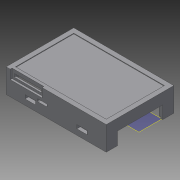
# Autodesk Inventor part: Boden
Saved by Autodesk Inventor 2014 (Build 180170000, 170)
## iProperties
Created: 2016-07-27
Part Number: Boden
Material: Generisch
Document SubType Name: Modeling
Designer: cem
Density: 1 g/cm^3
Appearance: Vorgabe
Author: cem
Autodesk Inventor part; units mm, degrees
ref_plane "YZ Plane" through (0, 0, 0) normal (1, 0, 0) x (0, 1, 0)
ref_plane "XZ Plane" through (0, 0, 0) normal (0, 1, 0) x (-1, 0, 0)
ref_plane "EbeneBoden" through (-11.5031, -4.6031, 1.9) normal (0, 0, 1) x (1, 0, 0)
ref_plane "EbeneWändeEnde" through (17.7, 4.9, -6.9) normal (0, 0, -1) x (-1, 0, 0)
sketch "SkizzeBoden" plane through (-11.5031, -4.6031, 1.9) normal (0, 0, 1) x (1, 0, 0)
  line L0 (-7.1969, 7.4031) -> (6.8031, 7.4031) projected
  line L1 (6.8031, 7.4031) -> (6.8031, -7.7969) projected
  line L2 (6.8031, -7.7969) -> (4.3031, -7.7969) projected
  line L3 (4.3031, -7.7969) -> (4.3031, -6.7969) projected
  line L4 (4.3031, -6.7969) -> (-7.1969, -6.7969) projected
  line L5 (-7.1969, -6.7969) -> (-7.1969, 7.4031) projected
  line L6 (31.5031, 17.6031) -> (-8.4969, 17.6031) projected
  line L7 (-8.4969, 17.6031) -> (-8.4969, -8.3969) projected
  line L8 (-8.4969, -8.3969) -> (31.5031, -8.3969) projected
  line L9 (31.5031, -8.3969) -> (31.5031, 17.6031) projected
  line L10 (-18.7369, 4.6031) -> (41.7431, 4.6031) projected
  line L11 (11.5031, -15.8369) -> (11.5031, 25.0431) projected
  line L12 (-10.0969, 19.2031) -> (33.1031, 19.2031)
  line L13 (33.1031, 19.2031) -> (33.1031, -9.9969)
  line L14 (33.1031, -9.9969) -> (-10.0969, -9.9969)
  line L15 (-10.0969, -9.9969) -> (-10.0969, 19.2031)
  point P0 (11.5031, 4.6031)
  dimension "d0" = 1.6
  constraints: 8 end point, 3 other
  measures "d0" distance between parallel lines of L7 L15
extrude "Boden" add sketch "SkizzeBoden" along normal blind 1.5
sketch "SkizzeWände" plane through (-11.5031, -4.6031, 1.9) normal (0, 0, -1) x (-1, 0, 0)
  line L0 (10.0969, 19.2031) -> (-33.1031, 19.2031) projected
  line L1 (-33.1031, 19.2031) -> (-33.1031, -9.9969) projected
  line L2 (-33.1031, -9.9969) -> (10.0969, -9.9969) projected
  line L3 (10.0969, -9.9969) -> (10.0969, 19.2031) projected
  line L4 (-31.6031, 17.7031) -> (8.5969, 17.7031)
  line L5 (8.5969, 17.7031) -> (8.5969, -8.4969)
  line L6 (8.5969, -8.4969) -> (-31.6031, -8.4969)
  line L7 (-31.6031, -8.4969) -> (-31.6031, 17.7031)
  point P0 (-11.5031, 4.6031)
  dimension "d3" = 1.5
  constraints: 8 end point, 3 other
  measures "d3" distance between parallel lines of L7 L1
extrude "Wände" add sketch "SkizzeWände" along normal up to surface (8.8 mm away)
sketch "SkizzeAuflage" plane through (-11.5031, -4.6031, 1.9) normal (0, 0, -1) x (-1, 0, 0)
  line L0 (8.5969, -8.4969) -> (8.5969, 17.7031) projected
  line L1 (-31.6031, -8.4969) -> (8.5969, -8.4969) projected
  line L2 (-31.6031, 17.7031) -> (-31.6031, -8.4969) projected
  line L3 (8.5969, 17.7031) -> (-31.6031, 17.7031) projected
  line L4 (10.0969, 19.2031) -> (10.0969, -9.9969) projected
  line L5 (-33.1031, 19.2031) -> (10.0969, 19.2031) projected
  line L6 (-33.1031, -9.9969) -> (-33.1031, 19.2031) projected
  line L7 (10.0969, -9.9969) -> (-33.1031, -9.9969) projected
  line L8 (-26.6031, 3.5031) -> (-25.1031, 3.5031)
  line L9 (-25.1031, 3.5031) -> (-25.1031, -6.4969)
  line L10 (-25.1031, -6.4969) -> (-26.6031, -6.4969)
  line L11 (-26.6031, -6.4969) -> (-26.6031, 3.5031)
  line L12 (-17.1031, 3.5031) -> (-15.6031, 3.5031)
  line L13 (-15.6031, 3.5031) -> (-15.6031, -6.4969)
  line L14 (-15.6031, -6.4969) -> (-17.1031, -6.4969)
  line L15 (-17.1031, -6.4969) -> (-17.1031, 3.5031)
  line L16 (6.5969, 13.7031) -> (-13.4031, 13.7031)
  line L17 (-13.4031, 13.7031) -> (-13.4031, 12.2031)
  line L18 (-13.4031, 12.2031) -> (6.5969, 12.2031)
  line L19 (6.5969, 12.2031) -> (6.5969, 13.7031)
  point P0 (-11.5031, 4.6031)
  dimension "d6" = 5
  dimension "d7" = 1.5
  dimension "d8" = 8
  dimension "d9" = 2
  dimension "d10" = 10
  dimension "d11" = 20
  dimension "d12" = 1.5
  dimension "d13" = 4
  dimension "d14" = 2
  constraints: 24 end point, 6 parallel, 3 horizontal, 3 perpendicular, 2 equal length, 1 collinear
  measures "d6" distance between parallel lines of L11 L2
  measures "d7" distance between parallel lines of L9 L11
  measures "d8" distance between parallel lines of L15 L9
  measures "d9" distance between parallel lines of L10 L1
  measures "d10" distance between parallel lines of L10 L8
  measures "d11" distance of L18.end L17.end
  measures "d12" distance of L17.end L16.end
  measures "d13" distance between parallel lines of L3 L16
  measures "d14" distance between parallel lines of L0 L19
ref_plane "EbeneAuflage" through (-20, -13, 0) normal (0, 0, 1) x (1, 0, 0)
extrude "Auflage" add sketch "SkizzeAuflage" along normal up to surface (1.9 mm away) contours L8 L9 L10 L11 | L12 L13 L14 L15 | L19 L18 L17 L16
sketch "SkizzeSD" plane through (-21.6, -14.6, 3.4) normal (0, -1, 0) x (1, 0, 0)
  line L0 (43.2, 0) -> (43.2, -10.3) projected
  line L1 (3.1, -2.6) -> (14.2, -2.6) projected
  line L2 (14.2, -2.6) -> (14.2, -1.6) projected
  line L3 (14.2, -1.6) -> (3.1, -1.6) projected
  line L4 (3.1, -1.6) -> (3.1, -2.6) projected
  line L5 (41.7, -1.5) -> (1.5, -1.5) projected
  line L6 (14.5, -1.5) -> (2.8, -1.5)
  line L7 (2.8, -1.5) -> (2.8, -2.9)
  line L8 (2.8, -2.9) -> (14.5, -2.9)
  line L9 (14.5, -2.9) -> (14.5, -1.5)
  line L10 (8.65, -4) -> (8.65, -0.8838) construction
  point P0 (21.6, -3.4)
  point P1 (8.65, -2.6)
  dimension "d17" = 0.3
  dimension "d18" = 0.3
  constraints: 10 end point, 4 parallel, 2 point on line, 1 horizontal, 1 midpoint, 1 perpendicular, 1 other
  measures "d17" distance between parallel lines of L8 L1
  measures "d18" distance between parallel lines of L7 L4
extrude "SD" cut sketch "SkizzeSD" against normal up to surface (1.5 mm away) contours L4 L3 L2 L1 | L9 L8 L7 L5
sketch "Skizze7" plane through (-21.6, -14.6, 3.4) normal (0, -1, 0) x (1, 0, 0)
  line L0 (14.5, -1.5) -> (14.5, -2.9) projected
  line L1 (14.5, -2.9) -> (2.8, -2.9) projected
  line L2 (0, 0) -> (43.2, 0) projected
  line L3 (15.5, -3.9) -> (1.8, -3.9)
  line L4 (1.8, -3.9) -> (1.8, 0)
  line L5 (1.8, 0) -> (15.5, 0)
  line L6 (15.5, 0) -> (15.5, -3.9)
  line L7 (8.65, -3.6567) -> (8.65, -1) construction
  point P0 (21.6, -3.4)
  point P1 (8.65, -2.9)
  dimension "d21" = 1
  dimension "d22" = 1
  constraints: 10 end point, 3 parallel, 1 collinear, 1 horizontal, 1 midpoint, 1 perpendicular, 1 point on line, 1 other
  measures "d21" distance between parallel lines of L3 L1
  measures "d22" distance between parallel lines of L0 L6
extrude "SDHilfe" cut sketch "Skizze7" against normal blind 0.8
sketch "SkizzeLED" plane through (-21.6, -14.6, -6.9) normal (0, -1, 0) x (1, 0, 0)
  line L0 (16.6, 5.2) -> (17.6, 5.2) projected
  line L1 (16.6, 5.2) -> (16.6, 4.1) projected
  line L2 (17.6, 4.1) -> (16.6, 4.1) projected
  line L3 (17.6, 5.2) -> (17.6, 4.1) projected
  line L4 (15.1, 5.2) -> (16.1, 5.2) projected
  line L5 (15.1, 5.2) -> (15.1, 4.1) projected
  line L6 (16.1, 4.1) -> (15.1, 4.1) projected
  line L7 (16.1, 5.2) -> (16.1, 4.1) projected
  line L8 (13.6, 5.2) -> (14.6, 5.2) projected
  line L9 (13.6, 5.2) -> (13.6, 4.1) projected
  line L10 (14.6, 4.1) -> (13.6, 4.1) projected
  line L11 (14.6, 5.2) -> (14.6, 4.1) projected
  line L12 (15.6, 3.5363) -> (15.6, 5.4531) construction
  line L13 (17.7, 4.1) -> (13.5, 4.1)
  line L14 (13.5, 4.1) -> (13.5, 5.2)
  line L15 (13.5, 5.2) -> (17.7, 5.2)
  line L16 (17.7, 5.2) -> (17.7, 4.1)
  line L17 (41.6, 5.2) -> (1.6, 5.2) projected
  point P0 (21.6, 6.9)
  point P1 (15.6, 4.1)
  dimension "d25" = 0.1
  constraints: 10 end point, 3 parallel, 2 collinear, 1 horizontal, 1 midpoint, 1 perpendicular, 1 point on line, 1 other
  measures "d25" distance between parallel lines of L3 L16
extrude "LED" cut sketch "SkizzeLED" against normal up to surface (1.5 mm away)
fillet "RundungLED" radius 0.3 4 edges at (-8.1, -13.85, -2.8) (-3.9, -13.85, -2.8) (-8.1, -13.85, -1.7) (-3.9, -13.85, -1.7)
sketch "SkizzeUSB" plane through (-21.6, 14.6, 3.4) normal (0, 1, 0) x (1, 0, 0)
  line L0 (43.2, 10.3) -> (0, 10.3) projected
  ellipse E0 centre (28.273, 7.641) end of major axis (28.5965, 8.1263) minor radius 0.5 (28.8, 7.72) -> (28.3475, 8.2) ccw projected
  line L1 (28.3475, 8.2) -> (21.3525, 8.2) projected
  ellipse E1 centre (21.427, 7.641) end of major axis (21.1035, 8.1263) minor radius 0.5 (21.3525, 8.2) -> (20.9, 7.72) ccw projected
  line L2 (20.9, 7.72) -> (20.9, 6.4602) projected
  line L3 (22.4652, 4.8) -> (20.9, 6.4602) projected
  line L4 (22.4652, 4.8) -> (27.2348, 4.8) projected
  line L5 (28.8, 6.4602) -> (27.2348, 4.8) projected
  line L6 (28.8, 6.4602) -> (28.8, 7.72) projected
  ellipse E2 centre (28.273, 7.641) end of major axis (28.5965, 8.1263) minor radius 0.5 (28.8, 7.72) -> (28.3475, 8.2) ccw projected
  line L7 (28.3475, 8.2) -> (21.3525, 8.2) projected
  ellipse E3 centre (21.427, 7.641) end of major axis (21.1035, 8.1263) minor radius 0.5 (21.3525, 8.2) -> (20.9, 7.72) ccw projected
  line L8 (20.9, 7.72) -> (20.9, 6.4602) projected
  line L9 (22.4652, 4.8) -> (20.9, 6.4602) projected
  line L10 (22.4652, 4.8) -> (27.2348, 4.8) projected
  line L11 (28.8, 6.4602) -> (27.2348, 4.8) projected
  line L12 (28.8, 6.4602) -> (28.8, 7.72) projected
  line L13 (20.6, 10.3) -> (29.1, 10.3)
  line L14 (29.1, 10.3) -> (29.1, 4.5)
  line L15 (29.1, 4.5) -> (20.6, 4.5)
  line L16 (20.6, 4.5) -> (20.6, 10.3)
  line L17 (24.85, 8.6856) -> (24.85, 4.4469) construction
  point P0 (21.6, 3.4)
  point P1 (24.85, 8.2)
  dimension "d29" = 0.3
  dimension "d30" = 0.3
  constraints: 10 end point, 3 parallel, 1 collinear, 1 horizontal, 1 midpoint, 1 perpendicular, 1 point on line, 5 other
  measures "d29" distance between parallel lines of L2 L16
  measures "d30" distance between parallel lines of L4 L15
extrude "USB" cut sketch "SkizzeUSB" against normal up to surface (1.5 mm away) contours L14 L15 L16 L0 | L6 L5 L4 L3 L2 E1 L1 E0
chamfer "FaseUSB" distance 1.5 angle 45 2 edges at (7.5, 13.85, -1.1) (-1, 13.85, -1.1)
sketch "Skizze10" plane through (-21.6, -14.6, 3.4) normal (-1, 0, 0) x (0, 0, 1)
  line L0 (-10.3, 29.2) -> (-10.3, 0) projected
  line L1 (-5.1, 27) -> (-5.1, 12) projected
  line L2 (-5.1, 27) -> (-8.8, 27) projected
  line L3 (-8.8, 12) -> (-8.8, 27) projected
  line L4 (-5.1, 12) -> (-8.8, 12) projected
  line L5 (-5.1, 11.2) -> (-5.1, 2.2) projected
  line L6 (-5.1, 11.2) -> (-8.8, 11.2) projected
  line L7 (-8.8, 2.2) -> (-8.8, 11.2) projected
  line L8 (-5.1, 2.2) -> (-8.8, 2.2) projected
  line L9 (-4.8, 1.9) -> (-10.3, 1.9)
  line L10 (-10.3, 1.9) -> (-10.3, 27.3)
  line L11 (-10.3, 27.3) -> (-4.8, 27.3)
  line L12 (-4.8, 27.3) -> (-4.8, 1.9)
  line L13 (0, 29.2) -> (0, 0) projected
  line L14 (-10.3, 29.2) -> (0, 29.2) projected
  line L15 (3, 14.6) -> (-13.529, 14.6) construction
  line L16 (-8.4, 2.6) -> (-8.4, 10.8) projected
  line L17 (-8.4, 10.8) -> (-5.5, 10.8) projected
  line L18 (-5.5, 10.8) -> (-5.5, 2.6) projected
  line L19 (-5.5, 2.6) -> (-8.4, 2.6) projected
  line L20 (-8.4, 12.4) -> (-8.4, 26.6) projected
  line L21 (-8.4, 26.6) -> (-5.5, 26.6) projected
  line L22 (-5.5, 26.6) -> (-5.5, 12.4) projected
  line L23 (-5.5, 12.4) -> (-8.4, 12.4) projected
  point P0 (-3.4, 14.6)
  point P1 (0, 14.6)
  dimension "d36" = 0.3
  dimension "d38" = 0.3
  constraints: 10 end point, 3 parallel, 1 collinear, 1 horizontal, 1 midpoint, 1 perpendicular, 1 point on line, 1 other
  measures "d36" distance between parallel lines of L8 L9
  measures "d38" distance between parallel lines of L5 L12
extrude "JSTFC" cut sketch "Skizze10" against normal up to surface (1.5 mm away) contours L11 L12 L9 L0 | L1 L4 L3 L2 | L5 L8 L7 L6 | L16 L17 L18 L19 | L20 L21 L22 L23
sketch "Skizze11" plane through (21.6, -14.6, 3.4) normal (1, 0, 0) x (0, 0, -1)
  line L0 (10.3, 0) -> (10.3, 29.2) projected
  line L1 (13.0125, 14.6) -> (-3.6442, 14.6) construction
  line L2 (5.1, 15) -> (5.1, 24) projected
  line L3 (5.1, 15) -> (8.8, 15) projected
  line L4 (8.8, 24) -> (8.8, 15) projected
  line L5 (5.1, 24) -> (8.8, 24) projected
  line L6 (5.1, 5.2) -> (5.1, 14.2) projected
  line L7 (5.1, 5.2) -> (8.8, 5.2) projected
  line L8 (8.8, 14.2) -> (8.8, 5.2) projected
  line L9 (5.1, 14.2) -> (8.8, 14.2) projected
  line L10 (10.3, 24.3) -> (4.8, 24.3)
  line L11 (4.8, 24.3) -> (4.8, 4.9)
  line L12 (4.8, 4.9) -> (10.3, 4.9)
  line L13 (10.3, 4.9) -> (10.3, 24.3)
  line L14 (5.5, 13.8) -> (8.4, 13.8) projected
  line L15 (8.4, 13.8) -> (8.4, 5.6) projected
  line L16 (8.4, 5.6) -> (5.5, 5.6) projected
  line L17 (5.5, 5.6) -> (5.5, 13.8) projected
  line L18 (8.4, 23.6) -> (8.4, 15.4) projected
  line L19 (8.4, 15.4) -> (5.5, 15.4) projected
  line L20 (5.5, 15.4) -> (5.5, 23.6) projected
  line L21 (5.5, 23.6) -> (8.4, 23.6) projected
  point P0 (3.4, 14.6)
  point P1 (10.3, 14.6)
  dimension "d41" = 0.3
  dimension "d42" = 0.3
  constraints: 10 end point, 2 parallel, 2 perpendicular, 1 collinear, 1 horizontal, 1 midpoint, 1 point on line, 1 other
  measures "d41" distance between parallel lines of L5 L10
  measures "d42" distance between parallel lines of L2 L11
extrude "JSTOSD" cut sketch "Skizze11" against normal up to surface (1.5 mm away) contours L12 L11 L10 L0 | L2 L5 L4 L3 | L6 L9 L8 L7 | L14 L15 L16 L17 | L18 L19 L20 L21
sketch "Skizze12" plane through (21.6, -14.6, -6.9) normal (0, 0, -1) x (-1, 0, 0)
  line L0 (0, 0) -> (0, 4.9) projected
  line L1 (43.2, 0) -> (0, 0) projected
  line L2 (21.6, -5.84) -> (21.6, 35.04) projected
  line L3 (51.84, 14.6) -> (-8.64, 14.6) projected
  line L4 (0.8, 28.4) -> (42.4, 28.4)
  line L5 (42.4, 28.4) -> (42.4, 0.8)
  line L6 (42.4, 0.8) -> (0.8, 0.8)
  line L7 (0.8, 0.8) -> (0.8, 28.4)
  point P0 (21.6, 14.6)
  dimension "d45" = 0.8
  dimension "d46" = 0.8
  constraints: 8 end point, 2 parallel, 1 horizontal, 1 perpendicular, 2 other
  measures "d45" distance between parallel lines of L1 L6
  measures "d46" distance between parallel lines of L0 L7
extrude "Lippe" cut sketch "Skizze12" against normal blind 0.6
sketch "SkizzeSchnapper" plane through (-21.6, -14.6, -6.9) normal (0, -1, 0) x (1, 0, 0)
  line L0 (36.2, 5.2) -> (41.6, 5.2) projected
  line L1 (36.2, 5.2) -> (36.2, 1.5) projected
  line L2 (42.4, 1.5) -> (36.2, 1.5) projected
  line L3 (42.4, 5.2) -> (42.4, 1.5) projected
  line L4 (41.6, 5.2) -> (42.4, 5.2) projected
  line L5 (0.8, 5.2) -> (1.6, 5.2) projected
  line L6 (0.8, 5.2) -> (0.8, 1.5) projected
  line L7 (7, 1.5) -> (0.8, 1.5) projected
  line L8 (7, 5.2) -> (7, 1.5) projected
  line L9 (1.6, 5.2) -> (7, 5.2) projected
  ellipse E0 centre (28.273, 2.659) end of major axis (28.5965, 2.1737) minor radius 0.5 (28.3475, 2.1) -> (28.8, 2.58) ccw projected
  line L10 (28.3475, 2.1) -> (21.3525, 2.1) projected
  ellipse E1 centre (21.427, 2.659) end of major axis (21.1035, 2.1737) minor radius 0.5 (20.9, 2.58) -> (21.3525, 2.1) ccw projected
  line L11 (20.9, 2.58) -> (20.9, 3.8398) projected
  line L12 (22.4652, 5.5) -> (20.9, 3.8398) projected
  line L13 (22.4652, 5.5) -> (27.2348, 5.5) projected
  line L14 (28.8, 3.8398) -> (27.2348, 5.5) projected
  line L15 (28.8, 3.8398) -> (28.8, 2.58) projected
  line L16 (35, 2.4) -> (30.5, 2.4)
  line L17 (30.5, 2.4) -> (30.5, 4)
  line L18 (30.5, 4) -> (35, 4)
  line L19 (35, 4) -> (35, 2.4)
  line L20 (21.6, -2.06) -> (21.6, 12.36) projected
  line L21 (1.5, 0.6) -> (0.8, 0.6) projected
  line L22 (41.7, 0.6) -> (1.5, 0.6) projected
  line L23 (42.4, 0.6) -> (41.7, 0.6) projected
  line L24 (0.8, 0.6) -> (42.4, 0.6) projected
  line L25 (41.6, 5.2) -> (1.6, 5.2) projected
  line L26 (8.2, 2.4) -> (12.7, 2.4)
  line L27 (12.7, 2.4) -> (12.7, 4)
  line L28 (12.7, 4) -> (8.2, 4)
  line L29 (8.2, 4) -> (8.2, 2.4)
  point P0 (21.6, 6.9)
  dimension "d49" = 4.5
  dimension "d50" = 1.8
  dimension "d51" = 1.2
  dimension "d52" = 1.6
  dimension "d53" = 1.2
  constraints: 16 end point, 4 symmetric about line, 2 parallel, 1 horizontal, 1 perpendicular, 2 other
  measures "d49" distance between parallel lines of L17 L19
  measures "d50" distance between parallel lines of L22 L16
  measures "d51" distance between parallel lines of L25 L18
  measures "d52" distance between parallel lines of L16 L18
  measures "d53" distance between parallel lines of L19 L1
extrude "Schnapper" cut sketch "SkizzeSchnapper" against normal up to surface (29.2 mm away) contours L16 L17 L18 L19 | L29 L28 L27 L26
sketch "SkizzeAufkleber" plane through (-11.5031, -4.6031, 3.4) normal (0, 0, 1) x (1, 0, 0)
  line L0 (33.1031, 19.2031) -> (-10.0969, 19.2031) projected
  line L1 (-10.0969, 19.2031) -> (-10.0969, -9.9969) projected
  line L2 (11.5031, -15.8369) -> (11.5031, 25.0431) projected
  line L3 (-18.7369, 4.6031) -> (41.7431, 4.6031) projected
  line L4 (-8.0969, 17.2031) -> (31.1031, 17.2031)
  line L5 (31.1031, 17.2031) -> (31.1031, -7.9969)
  line L6 (31.1031, -7.9969) -> (-8.0969, -7.9969)
  line L7 (-8.0969, -7.9969) -> (-8.0969, 17.2031)
  point P0 (11.5031, 4.6031)
  dimension "d56" = 2
  dimension "d57" = 2
  constraints: 8 end point, 2 parallel, 1 horizontal, 1 perpendicular, 2 other
  measures "d56" distance between parallel lines of L0 L4
  measures "d57" distance between parallel lines of L7 L1
extrude "Aufkleber" cut sketch "SkizzeAufkleber" against normal blind 0.3 contours L4 L5 L3 L2 | L2 L3 L7 L4 | L3 L5 L6 L2 | L2 L6 L7 L3
